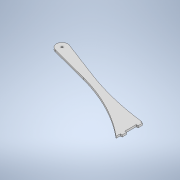
# Autodesk Inventor part: spray_holder_base
Saved by Autodesk Inventor 2020 (Build 240168000, 168)
## iProperties
Created: 2020-03-11
Part Number: spray_holder_base
Material: Generic
Document SubType Name: Modeling
Designer: erwin
Density: 1 g/cm^3
Appearance: Default
Author: erwin
Autodesk Inventor part; units mm, degrees
ref_plane "YZ Plane" through (0, 0, 0) normal (1, 0, 0) x (0, 1, 0)
ref_plane "XZ Plane" through (0, 0, 0) normal (0, 1, 0) x (-1, 0, 0)
ref_plane "XY Plane" through (0, 0, 0) normal (0, 0, 1) x (1, 0, 0)
sketch "Sketch1" plane through (0, 0, 0) normal (0, 1, 0) x (-1, 0, 0)
  line L0 (0, -5.0899) -> (4, -5.0899)
  line L1 (4, -5.0899) -> (4, 102.9101)
  line L2 (4, 102.9101) -> (0, 102.9101)
  line L3 (0, 102.9101) -> (0, -5.0899)
  line L4 (0, 102.9101) -> (-10, 102.9101)
  line L5 (-10, 102.9101) -> (-10, 78.9101)
  line L6 (-10, 78.9101) -> (0, 78.9101)
  line L7 (0, 78.9101) -> (0, 102.9101)
  line L8 (0, -5.0899) -> (-10, -5.0899)
  line L9 (-10, -5.0899) -> (-10, 18.9101)
  line L10 (-10, 18.9101) -> (0, 18.9101)
  line L11 (0, 18.9101) -> (0, -5.0899)
  circle A0 centre (550, -139.7792) radius 30
  line L12 (539.3198, -167.8136) -> (348.769, -95.22)
  line L13 (0, -5.0899) -> (0, -10.0899)
  arc A1 (348.769, -95.22) -> (0, -10.0899) centre (-165.497, -1445.1141) ccw
  line L14 (557.6456, -110.7698) -> (354.4922, -57.2275)
  arc A2 (0, 124.6706) -> (354.4922, -57.2275) centre (590.9573, 839.983) ccw
  line L15 (0, 124.6706) -> (0, 102.9101)
  point P0 (0, 0)
  dimension "d0" = 4
  dimension "d1" = 108
  dimension "d2" = 10
  dimension "d3" = 24
  dimension "d4" = 10
  dimension "d5" = 24
  dimension "d6" = 60
  dimension "d8" = 550
  constraints: 32 end point, 6 parallel, 6 point on circle, 4 tangent, 3 centre point, 3 horizontal, 3 perpendicular, 1 collinear, 1 point on line, 1 vertical
  measures "d0" distance of L2.end L1.end
  measures "d1" distance of L1.end L0.end
  measures "d2" distance of L6.end L5.end
  measures "d3" distance of L5.end L4.end
  measures "d4" distance of L9.end L10.end
  measures "d5" distance of L8.end L9.end
  measures "d6" diameter of A0
  measures "d8" distance from line of L3 A0.centre
extrude "Extrusion1" add sketch "Sketch1" along normal blind 10
sketch "Sketch2" plane through (0, 10, 0) normal (0, 1, 0) x (1, 0, 0)
  arc A0 (-539.3198, 167.8136) -> (-557.6456, 110.7698) centre (-550, 139.7792) ccw projected
  point P0 (0, 0)
  constraints: 1 coincident
hole "Hole1" at (-550, 10, -139.7792) direction (0, -1, 0) diameter 10 end through all
body "Solid1"
